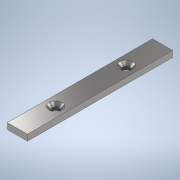
# Autodesk Inventor part: Parte5_BasePlaca_FMH
Saved by Autodesk Inventor 2021 (Build 250183000, 183)
## iProperties
Created: 2020-10-13
Part Number: Parte5_BasePlaca_FMH
Material: Steel, Alloy
Document SubType Name: Modeling
Designer: Fabia
Density: 7.73 g/cm^3
Appearance: Semi-Polished
Author: Fabia
Autodesk Inventor part; units mm, degrees
ref_plane "YZ Plane" through (0, 0, 0) normal (1, 0, 0) x (0, 1, 0)
ref_plane "XZ Plane" through (0, 0, 0) normal (0, 1, 0) x (-1, 0, 0)
ref_plane "XY Plane" through (0, 0, 0) normal (0, 0, 1) x (1, 0, 0)
sketch "Sketch1" plane through (0, 0, 0) normal (0, 1, 0) x (-1, 0, 0)
  line L0 (10, 72) -> (-10, 72)
  line L1 (-10, 72) -> (-10, -72)
  line L2 (-10, -72) -> (10, -72)
  line L3 (10, -72) -> (10, 72)
  line L4 (0, -72) -> (0, 72) construction
  circle A0 centre (0, 34) radius 3.5
  circle A1 centre (0, -36) radius 3.5
  point P0 (0, 0)
  point P1 (0, 0)
  dimension "d0" = 144
  dimension "d1" = 20
  dimension "d2" = 7
  dimension "d3" = 7
  dimension "d4" = 70
  dimension "d6" = 36
  dimension "d7" = 38
  constraints: 10 end point, 2 centre point, 2 midpoint, 2 parallel, 2 point on line, 1 coincident, 1 horizontal, 1 perpendicular
  measures "d0" distance of L0.end L1.end
  measures "d1" distance of L1.end L2.end
  measures "d2" diameter of A0
  measures "d3" diameter of A1
  measures "d4" distance of A0.centre A1.centre
  measures "d6" distance from line of L2 A1.centre
  measures "d7" distance from line of L0 A0.centre
extrude "Extrusion1" add sketch "Sketch1" against normal blind 6
chamfer "Chamfer1" distance 3 angle 45 2 edges at (3.5, 0, 34) (3.5, 0, -36)
body "Solid1"
